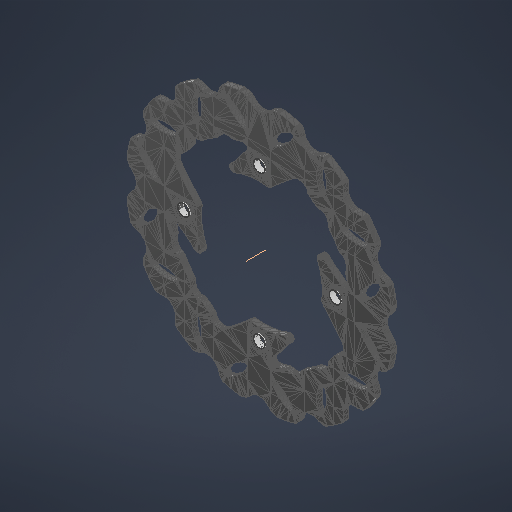
# Autodesk Inventor part: Arashi Rear Brake Disc Rotors
Saved by Autodesk Inventor 2026.1 (Build 301233000, 233)
## iProperties
Created: 2026-06-25
Part Number: Arashi Rear Brake Disc Rotors
Material: Generic
Document SubType Name: Modeling
Designer: share
Density: 1 g/cm^3
Appearance: Default
Author: share
Autodesk Inventor part; units mm, degrees
ref_plane "YZ Plane" through (0, 0, 0) normal (1, 0, 0) x (0, 1, 0)
ref_plane "XZ Plane" through (0, 0, 0) normal (0, 1, 0) x (-1, 0, 0)
ref_plane "XY Plane" through (0, 0, 0) normal (0, 0, 1) x (1, 0, 0)
sketch "Sketch1" plane through (19.2334, 117.838, 4.5) normal (0, 0, 1) x (1, 0, 0)
  circle A0 centre (102.3166, 4.662) radius 62.5 construction
  line L0 (-19.2334, 159.3689) -> (-19.2334, -164.0391) projected
  line L1 (-65.3026, -117.838) -> (257.1813, -117.838) projected
  line L2 (102.3166, 4.662) -> (102.3166, -57.838) construction
  circle A1 centre (102.3166, -57.838) radius 5
  line L3 (102.3166, 4.662) -> (102.3166, 67.162) construction
  circle A2 centre (102.3166, 67.162) radius 5
  line L4 (102.3166, 4.662) -> (39.8166, 4.662) construction
  circle A3 centre (39.8166, 4.662) radius 5
  line L5 (102.3166, 4.662) -> (164.8166, 4.662) construction
  circle A4 centre (164.8166, 4.662) radius 5
  circle A5 centre (102.3166, -57.838) radius 4.5
  circle A6 centre (39.8166, 4.662) radius 4.5
  circle A7 centre (102.3166, 67.162) radius 4.5
  circle A8 centre (164.8166, 4.662) radius 4.5
  point P0 (-19.2334, -117.838)
  dimension "d0" = 125
  dimension "d1" = 122.5
  dimension "d2" = 121.55
  dimension "d3" = 10
  dimension "d4" = 9
  constraints: 9 centre point, 8 coincident, 8 end point, 6 equal radius, 4 point on circle, 2 horizontal, 2 vertical
  measures "d0" diameter of A0
  measures "d1" distance from line of L1 L2.start
  measures "d2" distance from line of L0 L2.start
  measures "d3" diameter of A1
  measures "d4" diameter of A5
extrude "Extrusion1" add sketch "Sketch1" against normal blind 5
body "Solid1"
